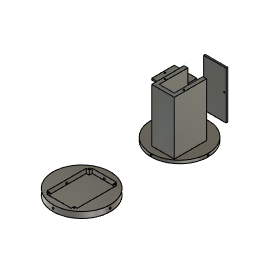
Attachments V1 (Autodesk Fusion 360 design; units mm, degrees)
Autodesk Fusion 360 part; units mm, degrees
note: some values were not read from the file. Chosen so that the rebuilt part matches the saved one: which bodies a step acts on; which face or edge a step refers to.
sketch "Sketch1" plane through (0, 0, 0) normal (0, 0, 1) x (1, 0, 0)
  circle A0 centre (0, 0) radius 38
  circle A1 centre (0, 0) radius 38.5
  dimension "d1" = 76
  dimension "d2" = 77
  constraint coincident A0.centre A1.centre
  measures "d1" diameter of A0
  measures "d2" diameter of A1
extrude "Extrude1" add sketch "Sketch1" along normal blind 230 makes body 1
copy_body "CutPasteBodies1" bodies 1 removing the originals makes body 2 in component "Rocket Body"
sketch "Sketch1 (2)" plane through (0, 0, 0) normal (0, 0, 1) x (1, 0, 0) in component "Battery holder"
  circle A0 centre (0, 0) radius 37.9
  dimension "d5" = 75.8
  constraint coincident A0.centre origin
  measures "d5" diameter of A0
extrude "Extrude1'" add sketch "Sketch1 (2)" along normal blind 4 separate body makes body 3 in component "Battery holder"
sketch "Sketch2" plane through (0, 0, 4) normal (0, 0, 1) x (-1, 0, 0) in component "Battery holder"
  circle A0 centre (0, 0) radius 37.9
  line L0 (10, -19) -> (-10, -19)
  line L1 (-10, -19) -> (-10, 19)
  line L2 (-10, 19) -> (10, 19)
  line L3 (10, 19) -> (10, -19)
  line L4 (10, -19) -> (10, -21)
  line L5 (10, -19) -> (12, -19)
  line L6 (-10, 19) -> (-12, 19)
  line L7 (-10, 19) -> (-10, 21)
  line L8 (-12, 21) -> (12, 21)
  line L9 (12, 21) -> (12, -21)
  line L10 (12, -21) -> (-12, -21)
  line L11 (-12, -21) -> (-12, 21)
  constraint horizontal L0
  constraint vertical L1
  constraint horizontal L2
  constraint vertical L3
  constraint perpendicular L0 L4
  constraint perpendicular L4 L5
  constraint perpendicular L1 L6
  constraint perpendicular L6 L7
  constraint horizontal L8
  constraint vertical L9
  constraint horizontal L10
  constraint vertical L11
extrude "Extrude2" add sketch "Sketch2" along normal blind 73 contours L0 L1 L4 L6 L10 L11 | L4 L5 L9 L10 | L2 L3 L5 L7 L8 L9 | L6 L7 L8 L11 bodies 3 in component "Battery holder"
sketch "Sketch3" plane through (0, 0, 77) normal (0, 0, 1) x (-1, 0, 0) in component "Battery holder"
  line L0 (-10, 19) -> (10, 19)
  line L1 (10, 19) -> (10, -19)
  line L2 (10, -19) -> (-10, -19)
  line L3 (-10, -19) -> (-10, 19)
  line L4 (-12, -21) -> (12, -21)
  line L5 (12, -21) -> (12, 21)
  line L6 (12, 21) -> (-12, 21)
  line L7 (-12, 21) -> (-12, -21)
  line L8 (12, -19) -> (10, -19)
  line L9 (-10, -19) -> (-12, -19)
  constraint coincident L5 L8.start
  constraint coincident L1.end L2.start
  constraint coincident L2.end L3.start
  constraint coincident L7 L9.end
  constraint perpendicular L7 L9
extrude "Extrude3" cut sketch "Sketch3" against normal blind 10 contours L2 L4 L5 L7 L8 L9 bodies 3 in component "Battery holder"
sketch "Sketch4" plane through (-10, 0, 0) normal (1, 0, 0) x (0, 1, 0) in component "Battery holder"
  line L0 (-19, 4) -> (19, 4)
  line L1 (19, 4) -> (19, 67)
  line L2 (19, 67) -> (19, 77)
  line L3 (19, 77) -> (-19, 77)
  line L4 (-19, 77) -> (-19, 4)
  line L5 (19, 77) -> (19, 75)
  line L6 (19, 75) -> (-19, 75)
  dimension "d16" = 2
  constraint coincident L2.end L3.start
  constraint coincident L2 L5.end
  constraint coincident L4 L6.end
  constraint perpendicular L4 L6
  measures "d16" distance of L2.end L5.end
extrude "Extrude4" add sketch "Sketch4" along normal up to surface (20 mm away) contours L2 L3 L4 L5 L6 bodies 3 in component "Battery holder"
extrude "Extrude5" add 1 faces at (-12, -7.6667, 49.3333) along direction (-1, 0, 0) blind 3 on bodies 3 bodies 3 in component "Battery holder"
extrude "Extrude6" add 1 faces at (12, -7.6667, 49.3333) along direction (1, 0, 0) blind 3 on bodies 3 bodies 3 in component "Battery holder"
extrude "Extrude7" add 1 faces at (5, -21, 52.6667) along direction (0, -1, 0) blind 3 on bodies 3 bodies 3 in component "Battery holder"
sketch "Sketch5" plane through (0, 21, 0) normal (0, 1, 0) x (-1, 0, 0) in component "Battery holder"
  line L0 (15, 67) -> (-15, 67)
  line L1 (-15, 67) -> (-15, 4)
  line L2 (-15, 4) -> (15, 4)
  line L3 (15, 4) -> (15, 67)
  line L4 (-15, 67) -> (-12.5, 67)
  line L5 (-12.5, 67) -> (-12.5, 38)
  circle A0 centre (-12.5, 38) radius 1
  dimension "d25" = 2.5
  dimension "d26" = 2
  constraint coincident L0.end L1.start
  constraint perpendicular L1 L4
  constraint perpendicular L4 L5
  constraint coincident L5.end A0.centre
  measures "d25" distance of L0.end L4.end
  measures "d26" diameter of A0
extrude "Extrude8" cut sketch "Sketch5" against normal blind 20 contours A0 bodies 3 in component "Battery holder"
sketch "Sketch6" plane through (0, 21, 0) normal (0, 1, 0) x (-1, 0, 0) in component "Battery holder"
  circle A0 centre (-12.5, 38) radius 1
  line L0 (15, 67) -> (-15, 67)
  line L1 (-15, 67) -> (-15, 4)
  line L2 (-15, 4) -> (15, 4)
  line L3 (15, 4) -> (15, 67)
  circle A1 centre (13, 38) radius 1
  dimension "d29" = 2
  measures "d29" diameter of A1
extrude "Extrude9" cut sketch "Sketch6" against normal blind 25 contours A1 bodies 3 in component "Battery holder"
split "Split1" by plane through (12, 19, 77) normal (0, 1, 0) bodies 3 makes body 4 at (4, 21, 15.0447) in component "Battery holder"
split "Split2" by plane through (0, 0, 4) normal (0, 0, 1) bodies 3 makes body 5 at (-15, -9.6667, 49.3333) in component "Battery holder"
split "Split3" by plane through (0, 0, 4) normal (0, 0, 1) bodies 4 makes body 6 at (4, 21, 15.0447) in component "Battery holder"
combine "Combine1" operation add target body 4 tool bodies 3 in component "Battery holder"
move_body "Move1" bodies 5 to x (1, 0, 0) y (0, 1, 0) z (0, 0, 1) at (7, -5, 0) in component "Battery holder"
move_face "OffsetFaces1" offset 3 5 faces at (19.4751, 14, 15.0009) (20.3333, 14, 73) (-5.6418, 14, 15.0009) (-4.3333, 14, 73) (-6, 14, 73.6667) on bodies 5 in component "Battery holder"
sketch "Sketch7" plane through (0, 0, 77) normal (0, 0, 1) x (-1, 0, 0) in component "Battery holder"
  line L0 (3, -17) -> (5, -17)
  line L1 (5, -17) -> (8, -17)
  line L2 (8, -17) -> (8, 29)
  line L3 (8, 29) -> (-22, 29)
  line L4 (-22, 29) -> (-22, -17)
  line L5 (-22, -17) -> (3, -17)
  line L6 (-22, -17) -> (-22, -16)
  line L7 (-22, -16) -> (8, -16)
  constraint coincident L4.end L5.start
  constraint coincident L4 L6.end
  constraint perpendicular L5 L6
  constraint coincident L2 L7.end
  constraint perpendicular L2 L7
extrude "Extrude10" cut sketch "Sketch7" against normal up to surface (73 mm away) contours L0 L1 L2 L4 L5 L6 L7 bodies 5 in component "Battery holder"
sketch "Sketch8" plane through (-8, 0, 0) normal (-1, 0, 0) x (0, -1, 0) in component "Battery holder"
  line L0 (-16, 77) -> (-16, 4)
  line L1 (-16, 4) -> (29, 4)
  line L2 (29, 4) -> (29, 77)
  line L3 (29, 77) -> (-16, 77)
sketch "Sketch9" plane through (0, 16, 0) normal (0, 1, 0) x (-1, 0, 0) in component "Battery holder"
  line L0 (-17, 4) -> (-17, 75)
  line L1 (-17, 75) -> (3, 75)
  line L2 (3, 75) -> (3, 4)
  line L3 (3, 4) -> (8, 4)
  line L4 (8, 4) -> (8, 77)
  line L5 (8, 77) -> (-22, 77)
  line L6 (-22, 77) -> (-22, 4)
  line L7 (-22, 4) -> (-17, 4)
  circle A0 centre (-19.5, 38) radius 1
  circle A1 centre (6, 38) radius 1
  line L8 (-17, 75) -> (-22, 75)
  line L9 (3, 75) -> (8, 75)
  constraint coincident L0.end L1.start
  constraint coincident L6 L8.end
  constraint perpendicular L6 L8
  constraint coincident L1.end L2.start
  constraint coincident L4 L9.end
  constraint perpendicular L4 L9
extrude "Extrude11" cut sketch "Sketch9" against normal blind 15 contours L1 L4 L5 L6 L8 L9 bodies 5 in component "Battery holder"
combine "Combine2" operation add target body 4 tool bodies 5 in component "Battery holder"
move_body "Move2" bodies 6 to x (1, 0, 0) y (0, 1, 0) z (0, 0, 1) at (0, 28, 0) in component "Battery holder"
sketch "Sketch10" plane through (17, 0, 0) normal (-1, 0, 0) x (0, -1, 0) in component "Battery holder"
  line L0 (-16, 75) -> (-16, 4)
  line L1 (-16, 4) -> (24, 4)
  line L2 (24, 4) -> (24, 75)
  line L3 (24, 75) -> (-1, 75)
  line L4 (-1, 75) -> (-16, 75)
  dimension "d37" = 40
  measures "d37" distance of L0 L2
move_face "OffsetFaces2" offset -2 2 faces at (19.5249, 16, 62.9991) (-5.6418, 16, 15.0009) on bodies 4 in component "Battery holder"
sketch "Sketch11" plane through (0, -24, 0) normal (0, 1, 0) x (-1, 0, 0) in component "Battery holder"
  line L0 (3, 75) -> (-17, 75)
  line L1 (-17, 75) -> (-17, 4)
  line L2 (-17, 4) -> (3, 4)
  line L3 (3, 4) -> (3, 75)
hole "Hole1" at (37.9, 0, 1.8966) direction (-1, 0, 0) diameter 2.4 depth 100 tip angle 180 bodies 4 in component "Battery holder"
hole "Hole2" at (0, -37.9, 2) direction (0, 1, 0) diameter 2.4 depth 100 tip angle 180 bodies 4 in component "Battery holder"
sketch "Sketch12" plane through (0, 49, 0) normal (0, 1, 0) x (-1, 0, 0) in component "Battery holder"
  circle A0 centre (13, 38) radius 1
  circle A1 centre (-12.5, 38) radius 1
  line L0 (15, 67) -> (-15, 67)
  line L1 (-15, 67) -> (-15, 4)
  line L2 (-15, 4) -> (15, 4)
  line L3 (15, 4) -> (15, 67)
sketch "Sketch13" plane through (0, 0, 77) normal (0, 0, 1) x (-1, 0, 0) in component "Battery holder"
  line L0 (-22, -1) -> (8, -1)
  line L1 (8, -1) -> (8, 29)
  line L2 (8, 29) -> (-22, 29)
  line L3 (-22, 29) -> (-22, -1)
  line L4 (2.901, -1) -> (2.901, 29)
  line L5 (8, 4.9795) -> (5.5, 4.9795)
  circle A0 centre (5.5, 14) radius 1
  line L6 (-22, 14) -> (-19.5, 14)
  circle A1 centre (-19.5, 14) radius 1
  dimension "d46" = 2.5
  dimension "d47" = 2
  dimension "d48" = 2.5
  dimension "d49" = 2
  constraint coincident L0 L4.start
  constraint coincident L2 L4.end
  constraint perpendicular L2 L4
  constraint coincident L1 L5.start
  constraint perpendicular L1 L5
  constraint midpoint L3 L6.start
  constraint perpendicular L3 L6
  constraint coincident L6.end A1.centre
  measures "d46" distance of L5.start L5.end
  measures "d47" diameter of A0
  measures "d48" distance of L6.start L6.end
  measures "d49" diameter of A1
extrude "Extrude12" cut sketch "Sketch13" against normal blind 25 contours A0 | A1 bodies 4 in component "Battery holder"
split "Split4" by plane through (-3, 16, 75) normal (0, 0, 1) bodies 4 makes body 7 at (3.0777, -3.7733, 77) in component "Battery holder"
move_body "Move3" bodies 7 to x (1, 0, 0) y (0, 1, 0) z (0, 0, 1) at (-50, 50, -45) in component "Battery holder"
sketch "Sketch1 (3)" plane through (0, 0, 0) normal (0, 0, 1) x (1, 0, 0) in component "PCB holder"
  circle A0 centre (0, -27.5) radius 1
  circle A1 centre (-35, -27.5) radius 1
  circle A2 centre (-35, 27.5) radius 1
  line L0 (-20, 30) -> (-40, 30)
  line L1 (-37.5, 27.5) -> (-37.5, 30)
  line L2 (-37.5, 30) -> (2.5, 30)
  line L3 (2.5, 30) -> (2.5, -30)
  line L4 (2.5, -30) -> (-37.5, -30)
  line L5 (-37.5, -30) -> (-37.5, 30)
  line L6 (-34, -27.5) -> (-35, -27.5)
  line L7 (-34, -27.5) -> (-37.5, -27.5)
  circle A3 centre (0, 27.5) radius 1
  dimension "d54" = 35
  dimension "d56" = 2
  dimension "d57" = 2
  dimension "d58" = 2
  dimension "d63" = 20
  dimension "d65" = 35
  dimension "d66" = 2
  constraint coincident A1.centre L6.end
  constraint coincident L0 L1.end
  constraint perpendicular L0 L1
  constraint horizontal L2
  constraint vertical L3
  constraint horizontal L4
  constraint vertical L5
  constraint coincident A1 L6.start
  measures "d54" distance of A1.centre A0.centre
  measures "d56" diameter of A0
  measures "d57" diameter of A1
  measures "d58" diameter of A2
  measures "d63" distance of L0.start L0.end
  measures "d65" distance of A2.centre A3.centre
  measures "d66" diameter of A3
extrude "Extrude1''" add sketch "Sketch1 (3)" along normal blind 1.5 separate body makes body 8 in component "PCB holder"
extrude "Extrude2'" add 1 faces at (-18.3333, -7.756, 0) along direction (0, 0, -1) blind 5 on bodies 8 bodies 8 in component "PCB holder"
move_body "Move1'" bodies 8 to x (1, 0, 0) y (0, 1, 0) z (0, 0, 1) at (20, 0, 0) in component "PCB holder"
sketch "Sketch2 (2)" plane through (-17.5, 0, 0) normal (-1, 0, 0) x (0, -1, 0) in component "PCB holder"
  line L0 (30, -5) -> (30, 1.5)
  line L1 (30, 1.5) -> (-30, 1.5)
  line L2 (-30, 1.5) -> (-30, -5)
  line L3 (-30, -5) -> (30, -5)
sketch "Sketch3 (2)" plane through (0, 30, 0) normal (0, 1, 0) x (-1, 0, 0) in component "PCB holder"
  line L0 (17.5, -5) -> (17.5, 1.5)
  line L1 (17.5, 1.5) -> (-22.5, 1.5)
  line L2 (-22.5, 1.5) -> (-22.5, -5)
  line L3 (-22.5, -5) -> (17.5, -5)
move_body "Move2'" bodies 8 to x (1, 0, 0) y (0, 1, 0) z (0, 0, 1) at (-2.5, 0, 0) in component "PCB holder"
sketch "Sketch4 (2)" plane through (0, 0, 0) normal (0, 0, 1) x (1, 0, 0) in component "PCB holder"
  circle A0 centre (0, 0) radius 37.9
  dimension "d71" = 75.8
  constraint coincident A0.centre origin
  measures "d71" diameter of A0
extrude "Extrude3'" add sketch "Sketch4 (2)" along normal blind 10 separate body makes body 9 in component "PCB holder"
move_body "Move3'" bodies 8 to x (1, 0, 0) y (0, 1, 0) z (0, 0, 1) at (0, 0, 35) in component "PCB holder"
extrude "Extrude4'" cut 1 faces at (5.6667, -8.878, 30) along direction (0, 0, -1) blind 26 on bodies 8 bodies 9 in component "PCB holder"
sketch "Sketch5 (2)" plane through (0, 0, 4) normal (0, 0, 1) x (-1, 0, 0) in component "PCB holder"
  circle A0 centre (-17.5, -27.5) radius 1
  circle A1 centre (17.5, -27.5) radius 1
  circle A2 centre (-17.5, 27.5) radius 1
  circle A3 centre (17.5, 27.5) radius 1
  line L0 (20, 30) -> (-20, 30)
  line L1 (-20, 30) -> (-20, -30)
  line L2 (-20, -30) -> (20, -30)
  line L3 (20, -30) -> (20, 30)
  line L4 (20, -25.0076) -> (15, -25.0076)
  line L5 (15, -25.0076) -> (15, -30)
  line L6 (-15, -30) -> (-15, -25)
  line L7 (-15, -25) -> (-20, -25)
  line L8 (-15, 25) -> (-20, 25)
  line L9 (-15, 25) -> (-15, 30)
  line L10 (20, 25) -> (15, 25)
  line L11 (15, 25) -> (15, 30)
  constraint coincident L3 L4.start
  constraint perpendicular L3 L4
  constraint coincident L2 L5.end
  constraint perpendicular L2 L5
  constraint coincident L2 L6.start
  constraint perpendicular L2 L6
  constraint coincident L1 L7.end
  constraint perpendicular L1 L7
  constraint coincident L1 L8.end
  constraint perpendicular L1 L8
  constraint perpendicular L8 L9
  constraint coincident L3 L10.start
  constraint perpendicular L3 L10
  constraint coincident L0 L11.end
  constraint perpendicular L0 L11
extrude "Extrude5'" add sketch "Sketch5 (2)" along normal blind 6 contours L0 L3 L10 L11 | L0 L1 L8 L9 | L2 L3 L4 L5 | L1 L2 L6 L7 bodies 9 in component "PCB holder"
sketch "Sketch6 (2)" plane through (0, 0, 30) normal (0, 0, -1) x (1, 0, 0) in component "PCB holder"
  circle A0 centre (17.5, -27.5) radius 1
  circle A1 centre (-17.5, -27.5) radius 1
  circle A2 centre (17.5, 27.5) radius 1
  circle A3 centre (-17.5, 27.5) radius 1
  line L0 (20, 30) -> (-20, 30)
  line L1 (-20, 30) -> (-20, -30)
  line L2 (-20, -30) -> (20, -30)
  line L3 (20, -30) -> (20, 30)
extrude "Extrude6'" cut sketch "Sketch6 (2)" along normal blind 37 contours A0 | A1 | A2 | A3 bodies 9 in component "PCB holder"
extrude "Extrude7'" cut 1 faces at (15, 28.3333, 6) along direction (1, 0, 0) blind 1 on bodies 9 bodies 9 in component "PCB holder"
extrude "Extrude8'" cut 1 faces at (17.3333, 25, 6) along direction (0, 1, 0) blind 1 on bodies 9 bodies 9 in component "PCB holder"
extrude "Extrude9'" cut 1 faces at (-18.3333, 25.0076, 6) along direction (0, 1, 0) blind 1 on bodies 9 bodies 9 in component "PCB holder"
extrude "Extrude10'" cut 1 faces at (-15, 27.3384, 6) along direction (-1, 0, 0) blind 1 on bodies 9 bodies 9 in component "PCB holder"
extrude "Extrude11'" cut 1 faces at (-15, -26.6667, 6) along direction (-1, 0, 0) blind 1 on bodies 9 bodies 9 in component "PCB holder"
extrude "Extrude12'" cut 1 faces at (-18.6667, -25, 6) along direction (0, -1, 0) blind 1 on bodies 9 bodies 9 in component "PCB holder"
extrude "Extrude13" cut 1 faces at (16.6667, -25, 6) along direction (0, -1, 0) blind 1 on bodies 9 bodies 9 in component "PCB holder"
extrude "Extrude14" cut 1 faces at (15, -27.3333, 6) along direction (1, 0, 0) blind 1 on bodies 9 bodies 9 in component "PCB holder"
extrude "Extrude15" cut 1 faces at (5.6667, -8.878, 0) along direction (0, 0, 1) blind 2 on bodies 9 bodies 9 in component "PCB holder"
hole "Hole1'" at (37.9, 0, 5.9708) direction (-1, 0, 0) diameter 2.4 depth 100 tip angle 180 bodies 9 in component "PCB holder"
hole "Hole2'" at (0, 37.9, 5.8755) direction (0, -1, 0) diameter 2.4 depth 100 tip angle 180 bodies 9 in component "PCB holder"
component "Rocket Body" placed x (1, 0, 0) y (0, 1, 0) z (0, 0, 1) at (0, 0, 0)
component "Battery holder" placed x (1, 0, 0) y (0, 1, 0) z (0, 0, 1) at (0, 0, 0)
component "PCB holder" placed x (1, 0, 0) y (0, 1, 0) z (0, 0, 1) at (0, 0, 0)
hidden bodies 8
